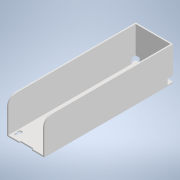
# Autodesk Inventor part: Hopper
Saved by Autodesk Inventor 2022 (Build 260153000, 153)
## iProperties
Created: 2022-01-17
Part Number: Hopper
Material: Generic
Document SubType Name: Modeling
Designer: Work
Density: 1 g/cm^3
Appearance: Default
Author: Work
Autodesk Inventor part; units mm, degrees
ref_plane "YZ Plane" through (0, 0, 0) normal (1, 0, 0) x (0, 1, 0)
ref_plane "XZ Plane" through (0, 0, 0) normal (0, 1, 0) x (-1, 0, 0)
ref_plane "XY Plane" through (0, 0, 0) normal (0, 0, 1) x (1, 0, 0)
sketch "Sketch1" plane through (0, 0, 0) normal (0, 0, 1) x (1, 0, 0)
  line L0 (0, 0) -> (87.28, 0)
  line L1 (0, 0) -> (0, 15.7)
  line L2 (87.28, 0) -> (87.28, 15.7)
  line L3 (87.28, 15.7) -> (0, 15.7)
  dimension "d0" = 87.28
  dimension "d1" = 15.7
  dimension "d2" = 15.7
  constraints: 8 end point, 2 vertical, 1 horizontal
  measures "d0" distance of L0.start L0.end
  measures "d1" distance of L0.start L1.end
  measures "d2" distance of L0.end L2.end
extrude "Extrusion1" add sketch "Sketch1" along normal blind 3
sketch "Sketch2" plane through (0, 0, 0) normal (0, -1, 0) x (1, 0, 0)
  line L0 (87.28, 0) -> (0, 0)
  line L1 (0, 0) -> (0, -297.64)
  line L2 (0, -297.64) -> (87.28, -297.64)
  line L3 (87.28, -297.64) -> (87.28, 0)
  dimension "d5" = 297.64
  constraints: 8 end point, 2 coincident, 2 parallel, 1 horizontal, 1 perpendicular
  measures "d5" distance of L1.end L0.end
extrude "Extrusion2" add sketch "Sketch2" against normal blind 3
sketch "Sketch3" plane through (87.28, 0, 3) normal (1, 0, 0) x (0, 0, -1)
  line L0 (0, 15.7) -> (0, 79.2)
  line L1 (0, 79.2) -> (3, 79.2)
  line L2 (3, 15.7) -> (0, 15.7) projected
  line L3 (3, 79.2) -> (3, 15.7)
  line L4 (3, 3) -> (3, 15.7) projected
  line L5 (3, 15.7) -> (3, 3)
  line L6 (3, 3) -> (300.64, 3)
  line L7 (300.64, 3) -> (300.64, 79.2)
  line L8 (300.64, 79.2) -> (3, 79.2)
  point P0 (3, 0)
  dimension "d8" = 63.5
  constraints: 14 end point, 4 perpendicular, 2 vertical, 1 coincident, 1 horizontal
  measures "d8" distance of L0.start L0.end
extrude "Extrusion3" add sketch "Sketch3" against normal blind 3
fillet "Fillet1" radius 20 1 edges at (85.78, 79.2, 3)
sketch "Sketch4" plane through (0, 0, 3) normal (-1, 0, 0) x (0, 0, 1)
  line L0 (0, 0) -> (0, 59.2) projected
  line L1 (0, 15.7) -> (0, 79.2)
  line L2 (0, 79.2) -> (-3, 79.2)
  line L3 (0, 15.7) -> (-3, 15.7) projected
  line L4 (-3, 79.2) -> (-3, 15.7)
  line L5 (-3, 15.7) -> (-3, 3) projected
  line L6 (-3, 15.7) -> (-3, 3)
  line L7 (-3, 3) -> (-300.64, 3)
  line L8 (-300.64, 0) -> (-300.64, 79.2) projected
  line L9 (-300.64, 79.2) -> (-300.64, 3)
  line L10 (-300.64, 79.2) -> (-3, 79.2)
  point P0 (-3, 0)
  dimension "d12" = 63.5
  dimension "d13" = 3
  constraints: 14 end point, 2 collinear, 2 perpendicular, 2 point on line, 1 horizontal, 1 vertical
  measures "d12" distance of L1.start L1.end
  measures "d13" distance of L1.end L2.end
extrude "Extrusion4" add sketch "Sketch4" against normal blind 3
fillet "Fillet2" radius 20 1 edges at (1.5, 79.2, 3)
sketch "Sketch5" plane through (87.28, 0, -297.64) normal (0, 0, -1) x (-1, 0, 0)
  line L0 (0, 79.2) -> (3, 79.2) projected
  line L1 (3, 3) -> (84.28, 3) projected
  line L2 (3, 79.2) -> (84.28, 79.2)
  line L3 (84.28, 79.2) -> (84.28, 3)
  line L4 (84.28, 3) -> (3, 3)
  line L5 (3, 3) -> (3, 79.2)
  point P0 (87.28, 0)
  constraints: 8 end point, 2 parallel, 1 horizontal, 1 perpendicular
extrude "Extrusion5" add sketch "Sketch5" against normal blind 3
sketch "Sketch6" plane through (87.28, 0, 3) normal (1, 0, 0) x (0, 0, -1)
  line L0 (300.64, 0) -> (300.64, 79.2) projected
  line L1 (300.64, 3) -> (288.125, 3)
  line L2 (300.64, 0) -> (0, 0) projected
  line L3 (300.64, 3) -> (300.64, 15.7)
  line L4 (288.125, 3) -> (288.125, 15.7)
  line L5 (288.125, 15.7) -> (300.64, 15.7)
  point P0 (3, 0)
  dimension "d19" = 3
  dimension "d20" = 12.515
  dimension "d21" = 12.7
  constraints: 8 end point, 2 horizontal, 2 point on line, 1 vertical
  measures "d19" distance between parallel lines of L2 L1
  measures "d20" distance of L1.start L1.end
  measures "d21" distance of L1.start L3.end
extrude "Extrusion6" cut sketch "Sketch6" against normal blind 3
sketch "Sketch7" plane through (87.28, 0, -297.64) normal (0, 0, -1) x (-1, 0, 0)
  line L0 (0, 15.7) -> (3, 15.7) projected
  line L1 (3, 15.7) -> (12.515, 15.7)
  line L2 (3, 15.7) -> (84.28, 15.7) projected
  line L3 (12.515, 15.7) -> (12.515, 3)
  line L4 (3, 3) -> (84.28, 3) projected
  line L5 (0, 3) -> (3, 3) projected
  line L6 (3, 3) -> (12.515, 3)
  line L7 (3, 15.7) -> (3, 3) projected
  line L8 (3, 15.7) -> (3, 3)
  point P0 (87.28, 0)
  dimension "d24" = 9.515
  constraints: 8 end point, 2 point on line, 1 collinear, 1 perpendicular, 1 vertical
  measures "d24" distance of L0.end L1.end
extrude "Extrusion7" cut sketch "Sketch7" against normal blind 3
sketch "Sketch8" plane through (87.28, 0, -297.64) normal (0, 0, -1) x (-1, 0, 0)
  line L0 (87.28, 0) -> (87.28, 79.2) projected
  line L1 (87.28, 3) -> (74.765, 3)
  line L2 (87.28, 0) -> (0, 0) projected
  line L3 (74.765, 3) -> (74.765, 15.7)
  line L4 (74.765, 15.7) -> (87.28, 15.7)
  line L5 (87.28, 15.7) -> (87.28, 3)
  dimension "d27" = 3
  dimension "d28" = 12.515
  dimension "d29" = 12.7
  constraints: 8 end point, 2 point on line, 1 collinear, 1 horizontal, 1 perpendicular, 1 vertical
  measures "d27" distance between parallel lines of L2 L1
  measures "d28" distance of L1.start L1.end
  measures "d29" distance of L1.end L3.end
extrude "Extrusion8" cut sketch "Sketch8" against normal blind 3
sketch "Sketch9" plane through (0, 0, -297.64) normal (-1, 0, 0) x (0, 0, 1)
  line L0 (0, 15.7) -> (3, 15.7) projected
  line L1 (3, 3) -> (3, 15.7) projected
  line L2 (3, 15.7) -> (3, 3)
  line L3 (12.515, 15.7) -> (0, 15.7) projected
  line L4 (3, 15.7) -> (12.515, 15.7)
  line L5 (12.515, 15.7) -> (12.515, 3) projected
  line L6 (12.515, 15.7) -> (12.515, 3)
  line L7 (12.515, 3) -> (3, 3)
  point P0 (297.64, 0)
  constraints: 8 end point, 2 collinear, 1 perpendicular, 1 vertical
extrude "Extrusion9" cut sketch "Sketch9" against normal blind 3
sketch "Sketch11" plane through (0, 3, 0) normal (0, 1, 0) x (1, 0, 0)
  line L0 (-15, 37) -> (-15, -63) projected
  line L1 (-15, -63) -> (35, -63) projected
  line L2 (35, -63) -> (35, 37) projected
  line L3 (35, 37) -> (-15, 37) projected
  line L4 (7, 7) -> (7, 13) projected
  arc A0 (13, 13) -> (7, 13) centre (10, 17) ccw projected
  line L5 (13, 13) -> (13, 7) projected
  arc A1 (7, 7) -> (13, 7) centre (10, 7) ccw projected
  line L6 (7, -48) -> (7, -42) projected
  arc A2 (13, -42) -> (7, -42) centre (10, -38) ccw projected
  line L7 (13, -42) -> (13, -48) projected
  arc A3 (7, -48) -> (13, -48) centre (10, -48) ccw projected
  line L8 (12.5, 7) -> (12.5, 13.2583)
  arc A4 (12.5, 13.2583) -> (7.5, 13.2583) centre (10, 17) ccw
  line L9 (7.5, 13.2583) -> (7.5, 7)
  arc A5 (7.5, 7) -> (12.5, 7) centre (10, 7) ccw
  point P0 (0, 0)
  dimension "d53" = 0.5
  constraints: 4 end point, 4 point on circle, 2 centre point, 3 other
  measures "d53" radial gap between concentric circles of A1 A5
extrude "Extrusion11" cut sketch "Sketch11" against normal blind 3 contours A5 L9 A4 L8
sketch "Sketch12" plane through (0, 3, 0) normal (0, 1, 0) x (1, 0, 0)
  arc A0 (78.39, 280.32) -> (72.39, 280.32) centre (75.39, 284.32) ccw
  line L0 (78.39, 280.32) -> (78.39, 274.32)
  line L1 (72.39, 274.32) -> (72.39, 280.32)
  arc A1 (72.39, 274.32) -> (78.39, 274.32) centre (75.39, 274.32) ccw
  line L2 (77.89, 274.32) -> (77.89, 280.5783)
  arc A2 (77.89, 280.5783) -> (72.89, 280.5783) centre (75.39, 284.32) ccw
  line L3 (72.89, 280.5783) -> (72.89, 274.32)
  arc A3 (72.89, 274.32) -> (77.89, 274.32) centre (75.39, 274.32) ccw
  point P0 (0, 0)
  dimension "d52" = 0.5
  constraints: 8 end point, 8 point on circle, 4 centre point, 2 vertical, 11 other
  measures "d52" radial gap between concentric circles of A1 A3
extrude "Extrusion12" cut sketch "Sketch12" against normal blind 10 contours A3 L3 A2 L2
sketch "Sketch13" plane through (0, 0, 3) normal (0, 0, 1) x (1, 0, 0)
  line L0 (0, 59.2) -> (3, 59.2) projected
  line L1 (0, 0) -> (0, 59.2) projected
  line L2 (0, 0) -> (87.28, 0) projected
  line L3 (87.28, 0) -> (87.28, 59.2) projected
  line L4 (84.28, 59.2) -> (87.28, 59.2) projected
  line L5 (84.28, 15.7) -> (84.28, 59.2) projected
  line L6 (84.28, 15.7) -> (3, 15.7) projected
  line L7 (3, 59.2) -> (3, 15.7) projected
  line L8 (3, 15.7) -> (84.28, 15.7)
  line L9 (84.28, 15.7) -> (84.28, 3)
  line L10 (84.28, 3) -> (3, 3)
  line L11 (3, 3) -> (3, 15.7)
  line L12 (0, 0) -> (87.28, 0) projected
  line L13 (58.64, 0) -> (28.64, 0)
  line L14 (28.64, 0) -> (28.64, 3)
  line L15 (28.64, 3) -> (58.64, 3)
  line L16 (58.64, 3) -> (58.64, 0)
  dimension "d54" = 0
  dimension "d55" = 3
  dimension "d56" = 30
  dimension "d57" = 28.64
  constraints: 16 end point, 4 parallel, 2 horizontal, 2 perpendicular, 2 point on line
  measures "d54" distance between parallel lines of L5 L9
  measures "d55" distance between parallel lines of L2 L10
  measures "d56" distance of L13.start L13.end
  measures "d57" distance between parallel lines of L3 L16
extrude "Extrusion13" cut sketch "Sketch13" against normal blind 3 contours L6 L9 L10 L11 | L14 L10 L16 L2
body "Solid1"
